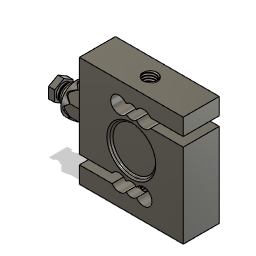
final test pad v3 (Autodesk Fusion 360 archive; units mm, degrees)
design "Untitled"
Autodesk Fusion 360 part; units mm, degrees
sketch "Sketch1" plane through (0, 0, 0) normal (0, 1, 0) x (1, 0, 0)
  line L0 (-17, 5.9) -> (17, 5.9)
  line L1 (17, 5.9) -> (17, -5.9)
  line L2 (17, -5.9) -> (-17, -5.9)
  line L3 (-17, -5.9) -> (-17, 5.9)
  line L4 (-17, 5.9) -> (17, -5.9) construction
  line L5 (17, 5.9) -> (-17, -5.9) construction
  dimension "d1" = 34
  dimension "d2" = 11.8
  constraint horizontal L0
  constraint perpendicular L0 L1
  constraint parallel L0 L2
  constraint parallel L1 L3
  constraint coincident L4 origin
  constraint coincident L5 origin
  measures "d1" distance of L1.end L2.end
  measures "d2" distance of L0.start L2.end
extrude "Extrude1" add sketch "Sketch1" along normal blind 36
sketch "Sketch2" plane through (0, 0, -5.9) normal (0, 0, -1) x (-1, 0, 0)
  line L0 (-17, 0) -> (17, 0)
  line L1 (17, 0) -> (17, 36)
  line L2 (17, 36) -> (-17, 36)
  line L3 (-17, 36) -> (-17, 0)
  line L4 (-17, 18) -> (17, 18) construction
  line L5 (0, 36) -> (0, 0) construction
  circle A0 centre (0, 18) radius 7.5
  circle A1 centre (0, 29) radius 2.25
  circle A2 centre (4, 29) radius 2.75
  circle A3 centre (-4, 29) radius 2.75
  line L6 (-6.3049, 30.5) -> (-17, 30.5)
  line L7 (-6.3049, 27.5) -> (-17, 27.5)
  line L8 (6.3049, 5.5) -> (17, 5.5)
  line L9 (6.3049, 8.5) -> (17, 8.5)
  circle A4 centre (4, 7) radius 2.75
  circle A5 centre (0, 7) radius 2.25
  circle A6 centre (-4, 7) radius 2.75
  dimension "d5" = 18
  dimension "d6" = 15
  dimension "d7" = 4.5
  dimension "d8" = 5.5
  dimension "d9" = 5.5
  dimension "d10" = 4
  dimension "d11" = 4
  dimension "d12" = 1.5
  dimension "d13" = 1.5
  dimension "d14" = 11
  dimension "d15" = 11
  dimension "d16" = 11
  dimension "d18" = 360
  constraint coincident L3 L4.start
  constraint perpendicular L3 L4
  constraint midpoint L2 L5.start
  constraint coincident L5.end origin
  constraint midpoint L5 A0.centre
  constraint coincident L5 A1.centre
  constraint coincident A3 L6.start
  constraint coincident L3 L6.end
  constraint perpendicular L3 L6
  constraint coincident A3 L7.start
  constraint coincident L3 L7.end
  constraint perpendicular L3 L7
  measures "d5" distance of L0 L4
  measures "d6" diameter of A0
  measures "d7" diameter of A1
  measures "d8" diameter of A2
  measures "d9" diameter of A3
  measures "d10" distance of A1.centre A3.centre
  measures "d11" distance of A1.centre A2.centre
  measures "d12" distance of A3.centre L6
  measures "d13" distance of A3.centre L7
  measures "d14" distance of A0.centre A1.centre
  measures "d15" distance of L4 A2.centre
  measures "d16" distance of L4 A3.centre
extrude "Extrude2" cut sketch "Sketch2" against normal blind 33 contours L3 A3 L6 L7 | L1 L8 L9 A4 | A1 A3 | A4 A5 | A1 A2 A3 | A1 A3 | A4 A5 A6 | A4 A5 | A1 A2 | A1 A2 | A5 A6 | A5 A6
extrude "Extrude3" cut sketch "Sketch2" against normal blind 1 contours A0
sketch "Sketch3" plane through (0, 0, 5.9) normal (0, 0, 1) x (1, 0, 0)
  line L0 (6.3049, 30.5) -> (17, 30.5)
  line L1 (17, 30.5) -> (17, 36)
  line L2 (17, 36) -> (-17, 36)
  line L3 (-17, 36) -> (-17, 8.5)
  line L4 (-17, 8.5) -> (-6.3049, 8.5)
  arc A0 (-1.6875, 8.4882) -> (-6.3049, 8.5) centre (-4, 7) ccw
  arc A1 (1.6875, 8.4882) -> (-1.6875, 8.4882) centre (0, 7) ccw
  arc A2 (1.6875, 5.5118) -> (1.6875, 8.4882) centre (4, 7) ccw
  arc A3 (-1.6875, 5.5118) -> (1.6875, 5.5118) centre (0, 7) ccw
  arc A4 (-6.3049, 5.5) -> (-1.6875, 5.5118) centre (-4, 7) ccw
  line L5 (-6.3049, 5.5) -> (-17, 5.5)
  line L6 (-17, 5.5) -> (-17, 0)
  line L7 (-17, 0) -> (17, 0)
  line L8 (17, 0) -> (17, 27.5)
  line L9 (17, 27.5) -> (6.3049, 27.5)
  arc A5 (1.6875, 27.5118) -> (6.3049, 27.5) centre (4, 29) ccw
  arc A6 (-1.6875, 27.5118) -> (1.6875, 27.5118) centre (0, 29) ccw
  arc A7 (-1.6875, 30.4882) -> (-1.6875, 27.5118) centre (-4, 29) ccw
  arc A8 (1.6875, 30.4882) -> (-1.6875, 30.4882) centre (0, 29) ccw
  arc A9 (6.3049, 30.5) -> (1.6875, 30.4882) centre (4, 29) ccw
  circle A10 centre (0, 18) radius 7.5
  dimension "d23" = 15
  measures "d23" diameter of A10
extrude "Extrude4" cut sketch "Sketch3" against normal blind 1 contours A10
fillet "Fillet1" radius 0.5 2 edges at (-6.9925, 20.7121, 5.9) (6.9925, 20.7121, -5.9)
fillet "Fillet2" radius 0.5 2 edges at (6.9925, 20.7121, -4.9) (-6.9925, 20.7121, 4.9)
sketch "Sketch4" plane through (0, 0, 0) normal (0, 0, 1) x (1, 0, 0)
  line L0 (-17, 13) -> (-17, 23)
  line L1 (-17, 23) -> (-24, 23)
  line L2 (-24, 23) -> (-26, 21)
  line L3 (-26, 21) -> (-26, 18)
  line L4 (-26, 18) -> (-17, 18)
  constraint vertical L0
  constraint perpendicular L0 L1
  constraint perpendicular L1 L3
  constraint midpoint L0 L4.end
  constraint perpendicular L0 L4
revolve "Revolve1" add sketch "Sketch4" angle 360 about axis through (-26, 18, 0) along (1, 0, 0)
ref_plane "WorkPlane1" through (-22.5385, 21.5355, 3.5355) normal (0, 0.707107, 0.707107) x (0, 0.707107, -0.707107)
sketch "Sketch5" plane through (-22.5385, 21.5355, 3.5355) normal (0, 0.707107, 0.707107) x (0, 0.707107, -0.707107)
  line L0 (-2, 1.4615) -> (2, 1.4615)
  line L1 (2, 1.4615) -> (2, -5.5385)
  line L2 (2, -5.5385) -> (-2, -5.5385)
  line L3 (-2, -5.5385) -> (-2, 1.4615)
  line L4 (-10.8894, -5.5385) -> (8.556, -5.5385)
  line L5 (-5, 1.4615) -> (5, 1.4615)
  circle A0 centre (0, 0) radius 0.8
  line L6 (-2, -1.1767) -> (-0.5564, 0.5748)
  line L7 (0.5564, 0.5748) -> (2, -1.1767)
  dimension "d46" = 2
  dimension "d47" = 2
  dimension "d48" = 1.6
  constraint horizontal L0
  constraint vertical L1
  constraint horizontal L2
  constraint vertical L3
  constraint coincident L1.end L4
  constraint coincident L0.end L5
  constraint coincident A0.centre origin
  constraint coincident L3 L6.start
  constraint coincident A0 L6.end
  constraint coincident A0 L7.start
  constraint coincident L1 L7.end
  measures "d46" distance of A0.centre L3
  measures "d47" distance of A0.centre L1
  measures "d48" diameter of A0
sketch "Sketch6" plane through (-26, 0, 0) normal (-1, 0, 0) x (0, 0, 1)
  circle A0 centre (0, 18) radius 3
extrude "Extrude6" add sketch "Sketch6" along normal blind 1
fillet "Fillet3" radius 0.5 1 edges at (-27, 16.9152, -2.797)
extrude "Extrude7" add 1 faces at (-27, 17.3299, 0.7673) along direction (-1, 0, 0) blind 1
fillet "Fillet4" radius 0.5 1 edges at (-27, 18.904, -2.3308)
sketch "Sketch7" plane through (-28, 0, 0) normal (-1, 0, 0) x (0, 0, 1)
  circle A0 centre (0, 18) radius 2.5
  circle A1 centre (0, 18) radius 3.5
  line L0 (-0.0433, 21.4997) -> (3.0092, 19.7874)
  line L1 (-3.0525, 19.7123) -> (-0.0433, 21.4997)
  line L2 (-3.0092, 16.2126) -> (-3.0525, 19.7123)
  line L3 (0.0433, 14.5003) -> (-3.0092, 16.2126)
  line L4 (3.0525, 16.2877) -> (0.0433, 14.5003)
  line L5 (3.0092, 19.7874) -> (3.0525, 16.2877)
  dimension "d61" = 7
  dimension "d65" = 360
  constraint concentric A0 A1
  constraint coincident A1 L0.start
  constraint coincident A1 L0.end
  measures "d61" diameter of A1
extrude "Extrude9" add sketch "Sketch7" along normal blind 2 contours A0 | L0 L1 L2 L3 L4 L5
extrude "Extrude10" cut sketch "Sketch5" against normal blind 0.5 contours L1 L2 L3 L4 A0 L6 L7 | A0 L6 L7
pattern_circular "C-Pattern2" count 8 over 360 about axis through (-31, 18, 0) along (1, 0, 0) of "Extrude10"
sketch "Sketch8" plane through (0, 0, 0) normal (0, -1, 0) x (1, 0, 0)
  line L0 (17, 5.9) -> (-17, 5.9)
  line L1 (-17, 5.9) -> (-17, -5.9)
  line L2 (-17, -5.9) -> (17, -5.9)
  line L3 (17, -5.9) -> (17, 5.9)
  circle A0 centre (0, 0) radius 1.75
  dimension "d72" = 3.5
  constraint coincident A0.centre origin
  measures "d72" diameter of A0
extrude "Extrude11" cut sketch "Sketch8" against normal blind 7 contours A0
thread "Thread3" "ISO Metric profile 5.0 M5x0.8 6H" major diameter 5.12 minor diameter 4.234 pitch 0.8 angle 60 modelled right hand crest width 0.2219 on face at (-1.7049, 1.8296, -0.3947) crest through (2.117, 0.2, 0)
sketch "Sketch9" plane through (0, 36, 0) normal (0, 1, 0) x (-1, 0, 0)
  line L0 (17, 5.9) -> (-17, 5.9)
  line L1 (-17, 5.9) -> (-17, -5.9)
  line L2 (-17, -5.9) -> (17, -5.9)
  line L3 (17, -5.9) -> (17, 5.9)
  circle A0 centre (0, 0) radius 1.75
  dimension "d75" = 3.5
  constraint coincident A0.centre origin
  measures "d75" diameter of A0
extrude "Extrude12" cut sketch "Sketch9" against normal blind 7 contours A0
thread "Thread4" "ISO Metric profile 5.0 M5x0.8 6H" major diameter 5.12 minor diameter 4.234 pitch 0.8 angle 60 modelled right hand crest width 0.2219 on face at (1.7049, 34.1704, -0.3947) crest through (-2.117, 35.8, 0)
